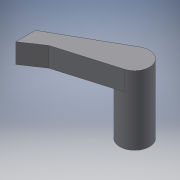
# Autodesk Inventor part: Pawl
Saved by Autodesk Inventor 2019 (Build 230136000, 136)
## iProperties
Created: 2019-08-06
Part Number: Pawl
Material: Generic
Document SubType Name: Modeling
Designer: aorfi
Density: 1 g/cm^3
Appearance: Default
Author: aorfi
Autodesk Inventor part; units mm, degrees
ref_plane "YZ Plane" through (0, 0, 0) normal (1, 0, 0) x (0, 1, 0)
ref_plane "XZ Plane" through (0, 0, 0) normal (0, 1, 0) x (-1, 0, 0)
ref_plane "XY Plane" through (0, 0, 0) normal (0, 0, 1) x (1, 0, 0)
sketch "Sketch1" plane through (0, 0, 0) normal (0, 1, 0) x (-1, 0, 0)
  circle A0 centre (0, 0) radius 1.5
  line L0 (0.74, -1.3048) -> (7.523, 2.5423)
  line L1 (5.523, 3.1933) -> (-0.4244, 1.4387)
  line L2 (5.523, 3.1933) -> (7.523, 4.5423)
  line L3 (7.523, 4.5423) -> (7.523, 2.5423)
  line L4 (7.523, 3.5) -> (7.523, 4.5) projected
  line L5 (7.4579, 4.5004) -> (6.1505, 3.6591) projected
  point P0 (7.523, 3.5423)
  dimension "d2" = 3
  dimension "d4" = 2
  dimension "d7" = 7.523
  dimension "d8" = 4.5423
  dimension "d9" = 56
  dimension "d10" = 2
  constraints: 8 end point, 2 point on circle, 2 tangent, 1 centre point, 1 coincident, 1 midpoint, 1 vertical
  measures "d2" diameter of A0
  measures "d4" distance of L2.end L0.end
  measures "d7" distance from line of L3 A0.centre
  measures "d8" vertical distance of L2.end A0.centre
  measures "d9" angle of L3 L2
  measures "d10" horizontal distance of L2.end L1.start
extrude "Extrusion1" add sketch "Sketch1" along normal mid plane 2
sketch "Sketch2" plane through (0, -1, 0) normal (0, 1, 0) x (1, 0, 0)
  arc A0 (0.4244, -1.4387) -> (-0.74, 1.3048) centre (0, 0) ccw projected
  circle A1 centre (0, 0) radius 1.5
  constraints: 1 centre point, 1 coincident, 1 concentric
extrude "Extrusion2" add sketch "Sketch2" against normal blind 5
body "Solid1"
